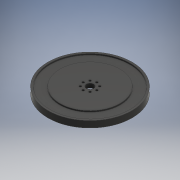
# Autodesk Inventor part: CS03
Saved by Autodesk Inventor 2017 (Build 210142000, 142)
## iProperties
Created: 2019-11-06
Part Number: CS03
Material: ABS Plastic
Document SubType Name: Modeling
Designer: Dell
Density: 1.06 g/cm^3
Appearance: Smooth - Black
Author: Dell
Autodesk Inventor part; units mm, degrees
ref_plane "YZ Plane" through (0, 0, 0) normal (1, 0, 0) x (0, 1, 0)
ref_plane "XZ Plane" through (0, 0, 0) normal (0, 1, 0) x (-1, 0, 0)
ref_plane "XY Plane" through (0, 0, 0) normal (0, 0, 1) x (1, 0, 0)
sketch "Sketch1" plane through (0, 0, 0) normal (0, 0, 1) x (1, 0, 0)
  circle A0 centre (0, 0) radius 40.5
  circle A1 centre (0, 0) radius 55.5
  dimension "d0" = 81
  dimension "d1" = 111
  constraints: 2 centre point, 2 coincident
  measures "d0" diameter of A0
  measures "d1" diameter of A1
extrude "Extrusion1" add sketch "Sketch1" along normal blind 7 contours A0 | A1
sketch "Sketch2" plane through (0, 0, 7) normal (0, 0, 1) x (1, 0, 0)
  circle A0 centre (0, 0) radius 55.5 projected
  circle A1 centre (0, 0) radius 53
  dimension "d4" = 106
  constraints: 1 centre point, 1 coincident
  measures "d4" diameter of A1
extrude "Extrusion2" add sketch "Sketch2" along normal blind 1.5
chamfer "Chamfer1" distance 1.5 angle 15 1 edges at (-53, 0, 7) measured on face at (-53, 0, 7.5)
sketch "Sketch3" plane through (0, 0, 7) normal (0, 0, 1) x (1, 0, 0)
  circle A0 centre (0, 0) radius 5
  dimension "d10" = 10
  constraints: 1 centre point, 1 coincident
  measures "d10" diameter of A0
extrude "Extrusion3" cut sketch "Sketch3" against normal through all
sketch "Sketch4" plane through (0, 0, 7) normal (0, 0, 1) x (1, 0, 0)
  circle A0 centre (0, 0) radius 5 projected
  circle A1 centre (0, 0) radius 39.5
  dimension "d13" = 79
  constraints: 1 centre point, 1 coincident
  measures "d13" diameter of A1
extrude "Extrusion4" add sketch "Sketch4" along normal blind 1.5
sketch "Sketch5" plane through (0, 0, 8.5) normal (0, 0, 1) x (1, 0, 0)
  circle A0 centre (9, 0) radius 1.5
  circle A1 centre (6.364, 6.364) radius 1.5
  circle A2 centre (0, 9) radius 1.5
  circle A3 centre (-6.364, 6.364) radius 1.5
  circle A4 centre (-9, 0) radius 1.5
  circle A5 centre (-6.364, -6.364) radius 1.5
  circle A6 centre (0, -9) radius 1.5
  circle A7 centre (6.364, -6.364) radius 1.5
  point P0 (0, 0)
  dimension "d16" = 3
  dimension "d17" = 9
  dimension "d20" = 360
  constraints: 8 centre point, 1 horizontal alignment, 17 other
  measures "d16" diameter of A0
  measures "d17" distance of A0.centre point (0, 0)
extrude "Extrusion5" cut sketch "Sketch5" against normal through all
chamfer "Chamfer2" distance 1.5 angle 15 1 edges at (-39.5, 0, 7) measured on face at (-39.5, 0, 7.5)
sketch "Sketch6" plane through (0, 0, 0) normal (0, 0, -1) x (-1, 0, 0)
  circle A0 centre (0, 9) radius 1.5 projected
  circle A1 centre (0, 9) radius 3.5
  circle A2 centre (0, 0) radius 12.5
  dimension "d27" = 7
  constraints: 2 centre point, 2 coincident, 1 tangent
  measures "d27" diameter of A1
extrude "Extrusion6" cut sketch "Sketch6" against normal blind 3 contours A0 | A1 | A2
body "Solid1"
